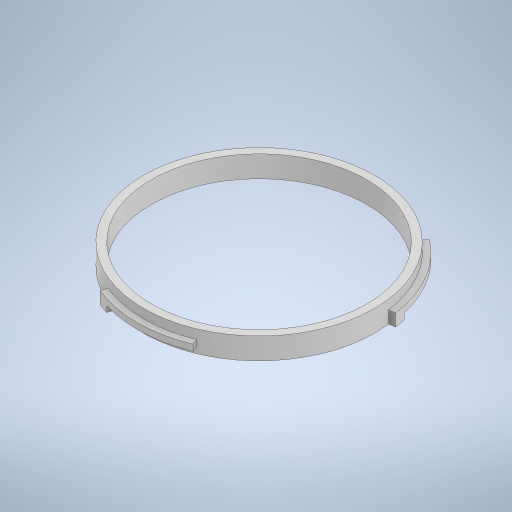
# Autodesk Inventor part: bottom_thread
Saved by Autodesk Inventor 2023 (Build 270158000, 158)
## iProperties
Created: 2025-12-29
Part Number: bottom_thread
Material: Generic
Document SubType Name: Modeling
Designer: Justin Pascual
Density: 1 g/cm^3
Appearance: Default
Author: Justin Pascual
Autodesk Inventor part; units mm, degrees
ref_plane "YZ Plane" through (0, 0, 0) normal (1, 0, 0) x (0, 1, 0)
ref_plane "XZ Plane" through (0, 0, 0) normal (0, 1, 0) x (-1, 0, 0)
ref_plane "XY Plane" through (0, 0, 0) normal (0, 0, 1) x (1, 0, 0)
sketch "Sketch1" plane through (0, 0, 0) normal (0, 1, 0) x (-1, 0, 0)
  circle A0 centre (0, 0) radius 47.625
  dimension "d0" = 95.25
  constraints: 1 centre point, 1 coincident
  measures "d0" diameter of A0
extrude "Extrusion1" add sketch "Sketch1" along normal blind 8.89
sketch "Sketch2" plane through (0, 8.89, 0) normal (0, 1, 0) x (1, 0, 0)
  circle A0 centre (0, 0) radius 44.45
  dimension "d3" = 88.9
  constraints: 1 centre point, 1 coincident
  measures "d3" diameter of A0
extrude "Extrusion2" cut sketch "Sketch2" against normal through all
sketch "Sketch4" plane through (0, 0, 0) normal (1, 0, 0) x (0, 1, 0)
  line L0 (0, 47.625) -> (8.89, 47.625) projected
  line L1 (0, 47.625) -> (2.54, 47.625)
  line L2 (2.54, 47.625) -> (2.54, 50.165)
  line L3 (2.54, 50.165) -> (5.08, 50.165)
  line L4 (5.08, 50.165) -> (5.08, 47.625)
  line L5 (5.08, 47.625) -> (2.54, 47.625)
  line L6 (-1.778, 0) -> (10.668, 0) projected
  point P0 (0, 0)
  dimension "d17" = 2.54
  dimension "d18" = 2.54
  dimension "d19" = 2.54
  constraints: 10 end point, 3 point on line, 2 perpendicular, 1 collinear, 1 vertical
  measures "d17" distance of L1.start L1.end
  measures "d18" distance of L1.end L2.end
  measures "d19" distance of L2.end L3.end
revolve "Revolution1" add sketch "Sketch4" angle 45 mid plane about axis through (0, -10, 0) along (0, 1, 0)
sketch "Sketch6" plane through (-19.1973, 2.54, 46.3464) normal (-0.9238795, 0, -0.3826834) x (-0.3826834, 0, 0.9238795)
  line L0 (-2.54, 0) -> (-2.54, 2.54) projected
  line L1 (-2.54, 0) -> (0, 0)
  line L2 (0, 0) -> (0, -2.54)
  line L3 (0, -2.54) -> (-2.54, -2.54)
  line L4 (-2.54, -2.54) -> (-2.54, 0)
  line L5 (-50.165, -4.318) -> (-50.165, 8.128) projected
  point P0 (-50.165, -2.54)
  dimension "d21" = 2.54
  dimension "d22" = 2.54
  constraints: 8 end point, 2 parallel, 1 horizontal, 1 perpendicular
  measures "d21" distance of L2.end L3.end
  measures "d22" distance of L1.end L2.end
revolve "Revolution2" add sketch "Sketch6" angle 5 about axis through (0, -10, 0) along (0, 1, 0)
fillet "Fillet3" radius 0.762 1 edges at (-14.703, 2.54, 46.632)
pattern_circular "Circular Pattern1" count 3 over 360 about axis through (0, -10, 0) along (0, 1, 0) of "Revolution1", "Revolution2", "Fillet3"
body "Solid1"
